Autodesk Inventor part; units mm, degrees
(part 2 of 2)
sketch "Sketch9" plane through (0, 0, 5.08) normal (0, 0, 1) x (1, 0, 0)
  arc A0 (133.35, 41.728) -> (148.59, 41.728) centre (140.97, 41.728) ccw projected
  line L0 (133.35, 41.728) -> (133.35, 92.528) projected
  arc A1 (148.59, 92.528) -> (133.35, 92.528) centre (140.97, 92.528) ccw projected
  line L1 (148.59, 92.528) -> (148.59, 41.728) projected
  line L2 (104.14, 0) -> (104.14, 5.08) projected
  line L3 (104.14, 5.08) -> (114.3, 5.08) projected
  line L4 (114.3, 5.08) -> (114.3, 0) projected
  line L5 (114.3, 0) -> (104.14, 0) projected
  line L6 (93.98, 5.08) -> (93.98, 0) projected
  line L7 (93.98, 0) -> (83.82, 0) projected
  line L8 (83.82, 0) -> (83.82, 5.08) projected
  line L9 (83.82, 5.08) -> (93.98, 5.08) projected
  line L10 (124.46, 0) -> (124.46, 5.08) projected
  line L11 (124.46, 5.08) -> (134.62, 5.08) projected
  line L12 (134.62, 5.08) -> (134.62, 0) projected
  line L13 (134.62, 0) -> (124.46, 0) projected
  line L14 (157.48, 65.405) -> (157.48, 55.245) projected
  line L15 (157.48, 55.245) -> (152.4, 55.245) projected
  line L16 (152.4, 55.245) -> (152.4, 65.405) projected
  line L17 (152.4, 65.405) -> (157.48, 65.405) projected
  line L18 (157.48, 45.085) -> (157.48, 34.925) projected
  line L19 (157.48, 34.925) -> (152.4, 34.925) projected
  line L20 (152.4, 34.925) -> (152.4, 45.085) projected
  line L21 (152.4, 45.085) -> (157.48, 45.085) projected
  line L22 (157.48, 24.765) -> (157.48, 14.605) projected
  line L23 (157.48, 14.605) -> (152.4, 14.605) projected
  line L24 (152.4, 14.605) -> (152.4, 24.765) projected
  line L25 (152.4, 24.765) -> (157.48, 24.765) projected
  line L26 (30.48, -80.01) -> (30.48, -90.17) projected
  line L27 (30.48, -90.17) -> (25.4, -90.17) projected
  line L28 (25.4, -90.17) -> (25.4, -80.01) projected
  line L29 (25.4, -80.01) -> (30.48, -80.01) projected
  line L30 (25.4, -59.69) -> (30.48, -59.69) projected
  line L31 (30.48, -59.69) -> (30.48, -69.85) projected
  line L32 (30.48, -69.85) -> (25.4, -69.85) projected
  line L33 (25.4, -69.85) -> (25.4, -59.69) projected
  line L34 (25.4, -39.37) -> (30.48, -39.37) projected
  line L35 (30.48, -39.37) -> (30.48, -49.53) projected
  line L36 (30.48, -49.53) -> (25.4, -49.53) projected
  line L37 (25.4, -49.53) -> (25.4, -39.37) projected
  line L38 (129.54, 45.72) -> (124.46, 45.72) projected
  line L39 (124.46, 45.72) -> (124.46, 55.88) projected
  line L40 (124.46, 55.88) -> (129.54, 55.88) projected
  line L41 (129.54, 55.88) -> (129.54, 45.72) projected
  line L42 (129.54, 96.52) -> (129.54, 86.36) projected
  line L43 (129.54, 86.36) -> (124.46, 86.36) projected
  line L44 (124.46, 86.36) -> (124.46, 96.52) projected
  line L45 (124.46, 96.52) -> (129.54, 96.52) projected
  line L46 (129.54, 76.2) -> (129.54, 66.04) projected
  line L47 (129.54, 66.04) -> (124.46, 66.04) projected
  line L48 (124.46, 66.04) -> (124.46, 76.2) projected
  line L49 (124.46, 76.2) -> (129.54, 76.2) projected
  line L50 (129.54, 111.578) -> (210.82, 111.578) projected
  line L51 (129.54, 111.578) -> (129.54, 106.68) projected
  line L52 (129.54, 106.68) -> (124.46, 106.68) projected
  line L53 (124.46, 106.68) -> (124.46, 111.578) projected
  line L54 (0, 111.578) -> (124.46, 111.578) projected
  line L55 (0, 111.578) -> (0, 101.6) projected
  line L56 (0, 101.6) -> (5.08, 101.6) projected
  line L57 (5.08, 101.6) -> (5.08, 91.44) projected
  line L58 (5.08, 91.44) -> (0, 91.44) projected
  line L59 (0, 91.44) -> (0, 81.28) projected
  line L60 (0, 81.28) -> (5.08, 81.28) projected
  line L61 (5.08, 81.28) -> (5.08, 71.12) projected
  line L62 (5.08, 71.12) -> (0, 71.12) projected
  line L63 (0, 71.12) -> (0, 60.96) projected
  line L64 (0, 60.96) -> (5.08, 60.96) projected
  line L65 (5.08, 60.96) -> (5.08, 50.8) projected
  line L66 (5.08, 50.8) -> (0, 50.8) projected
  line L67 (0, 50.8) -> (0, 40.64) projected
  line L68 (0, 40.64) -> (5.08, 40.64) projected
  line L69 (5.08, 40.64) -> (5.08, 30.48) projected
  line L70 (5.08, 30.48) -> (0, 30.48) projected
  line L71 (0, 30.48) -> (0, 20.32) projected
  line L72 (0, 20.32) -> (5.08, 20.32) projected
  line L73 (5.08, 20.32) -> (5.08, 10.16) projected
  line L74 (5.08, 10.16) -> (0, 10.16) projected
  line L75 (0, 10.16) -> (0, 0) projected
  line L76 (0, 0) -> (20.32, -95.25) projected
  line L77 (20.32, -95.25) -> (42.545, -95.25) projected
  line L78 (42.545, -95.25) -> (147.32, 9.525) projected
  line L79 (147.32, 9.525) -> (169.545, 9.525) projected
  line L80 (169.545, 9.525) -> (215.9, 35.56) projected
  line L81 (215.9, 35.56) -> (215.9, 45.72) projected
  line L82 (215.9, 45.72) -> (210.82, 45.72) projected
  line L83 (210.82, 45.72) -> (210.82, 55.88) projected
  line L84 (210.82, 55.88) -> (215.9, 55.88) projected
  line L85 (215.9, 55.88) -> (215.9, 66.04) projected
  line L86 (215.9, 66.04) -> (210.82, 66.04) projected
  line L87 (210.82, 66.04) -> (210.82, 76.2) projected
  line L88 (210.82, 76.2) -> (215.9, 76.2) projected
  line L89 (215.9, 76.2) -> (215.9, 86.36) projected
  line L90 (215.9, 86.36) -> (210.82, 86.36) projected
  line L91 (210.82, 86.36) -> (210.82, 96.52) projected
  line L92 (210.82, 96.52) -> (215.9, 96.52) projected
  line L93 (215.9, 96.52) -> (215.9, 106.68) projected
  line L94 (215.9, 106.68) -> (210.82, 106.68) projected
  line L95 (210.82, 106.68) -> (210.82, 111.578) projected
  line L96 (140.97, 92.528) -> (185.42, 92.528) construction
  line L97 (140.97, 84.908) -> (185.42, 84.908)
  line L98 (185.42, 100.148) -> (140.97, 100.148)
  arc A2 (140.97, 100.148) -> (140.97, 84.908) centre (140.97, 92.528) ccw
  arc A3 (185.42, 84.908) -> (185.42, 100.148) centre (185.42, 92.528) ccw
  point P0 (163.195, 92.528)
  dimension "d79" = 44.45
  dimension "d83" = 7.62
  constraints: 8 end point, 4 point on circle, 4 tangent, 2 centre point, 1 horizontal, 1 midpoint, 1 parallel
  measures "d79" distance of L96.start L96.end
  measures "d83" radius of A2
extrude "Extrusion10" cut sketch "Sketch9" against normal blind 25.4 contours A1 L1 L97 A2 | L1 A1 L98 A3 L97
fillet "Fillet1" radius 7.62 1 edges at (148.59, 84.908, 2.54)
sketch "Sketch10" plane through (0, 0, 5.08) normal (0, 0, 1) x (1, 0, 0)
  arc A0 (156.21, 84.908) -> (148.59, 77.288) centre (156.21, 77.288) ccw projected
  line L0 (148.59, 77.288) -> (148.59, 41.728) projected
  arc A1 (133.35, 41.728) -> (148.59, 41.728) centre (140.97, 41.728) ccw projected
  line L1 (133.35, 41.728) -> (133.35, 92.528) projected
  arc A2 (140.97, 100.148) -> (133.35, 92.528) centre (140.97, 92.528) ccw projected
  line L2 (140.97, 100.148) -> (185.42, 100.148) projected
  arc A3 (185.42, 84.908) -> (185.42, 100.148) centre (185.42, 92.528) ccw projected
  line L3 (185.42, 84.908) -> (156.21, 84.908) projected
  line L4 (129.54, 111.578) -> (210.82, 111.578) projected
  line L5 (129.54, 111.578) -> (129.54, 106.68) projected
  line L6 (129.54, 106.68) -> (124.46, 106.68) projected
  line L7 (124.46, 106.68) -> (124.46, 111.578) projected
  line L8 (0, 111.578) -> (124.46, 111.578) projected
  line L9 (0, 111.578) -> (0, 101.6) projected
  line L10 (0, 101.6) -> (5.08, 101.6) projected
  line L11 (5.08, 101.6) -> (5.08, 91.44) projected
  line L12 (5.08, 91.44) -> (0, 91.44) projected
  line L13 (0, 91.44) -> (0, 81.28) projected
  line L14 (0, 81.28) -> (5.08, 81.28) projected
  line L15 (5.08, 81.28) -> (5.08, 71.12) projected
  line L16 (5.08, 71.12) -> (0, 71.12) projected
  line L17 (0, 71.12) -> (0, 60.96) projected
  line L18 (0, 60.96) -> (5.08, 60.96) projected
  line L19 (5.08, 60.96) -> (5.08, 50.8) projected
  line L20 (5.08, 50.8) -> (0, 50.8) projected
  line L21 (0, 50.8) -> (0, 40.64) projected
  line L22 (0, 40.64) -> (5.08, 40.64) projected
  line L23 (5.08, 40.64) -> (5.08, 30.48) projected
  line L24 (5.08, 30.48) -> (0, 30.48) projected
  line L25 (0, 30.48) -> (0, 20.32) projected
  line L26 (0, 20.32) -> (5.08, 20.32) projected
  line L27 (5.08, 20.32) -> (5.08, 10.16) projected
  line L28 (5.08, 10.16) -> (0, 10.16) projected
  line L29 (0, 10.16) -> (0, 0) projected
  line L30 (0, 0) -> (20.32, -95.25) projected
  line L31 (20.32, -95.25) -> (42.545, -95.25) projected
  line L32 (42.545, -95.25) -> (147.32, 9.525) projected
  line L33 (147.32, 9.525) -> (169.545, 9.525) projected
  line L34 (169.545, 9.525) -> (215.9, 35.56) projected
  line L35 (215.9, 35.56) -> (215.9, 45.72) projected
  line L36 (215.9, 45.72) -> (210.82, 45.72) projected
  line L37 (210.82, 45.72) -> (210.82, 55.88) projected
  line L38 (210.82, 55.88) -> (215.9, 55.88) projected
  line L39 (215.9, 55.88) -> (215.9, 66.04) projected
  line L40 (215.9, 66.04) -> (210.82, 66.04) projected
  line L41 (210.82, 66.04) -> (210.82, 76.2) projected
  line L42 (210.82, 76.2) -> (215.9, 76.2) projected
  line L43 (215.9, 76.2) -> (215.9, 86.36) projected
  line L44 (215.9, 86.36) -> (210.82, 86.36) projected
  line L45 (210.82, 86.36) -> (210.82, 96.52) projected
  line L46 (210.82, 96.52) -> (215.9, 96.52) projected
  line L47 (215.9, 96.52) -> (215.9, 106.68) projected
  line L48 (215.9, 106.68) -> (210.82, 106.68) projected
  line L49 (210.82, 106.68) -> (210.82, 111.578) projected
  line L50 (129.54, 76.2) -> (129.54, 66.04) projected
  line L51 (129.54, 66.04) -> (124.46, 66.04) projected
  line L52 (124.46, 66.04) -> (124.46, 76.2) projected
  line L53 (124.46, 76.2) -> (129.54, 76.2) projected
  line L54 (129.54, 96.52) -> (129.54, 86.36) projected
  line L55 (129.54, 86.36) -> (124.46, 86.36) projected
  line L56 (124.46, 86.36) -> (124.46, 96.52) projected
  line L57 (124.46, 96.52) -> (129.54, 96.52) projected
  line L58 (129.54, 45.72) -> (124.46, 45.72) projected
  line L59 (124.46, 45.72) -> (124.46, 55.88) projected
  line L60 (124.46, 55.88) -> (129.54, 55.88) projected
  line L61 (129.54, 55.88) -> (129.54, 45.72) projected
  line L62 (25.4, -39.37) -> (30.48, -39.37) projected
  line L63 (30.48, -39.37) -> (30.48, -49.53) projected
  line L64 (30.48, -49.53) -> (25.4, -49.53) projected
  line L65 (25.4, -49.53) -> (25.4, -39.37) projected
  line L66 (25.4, -59.69) -> (30.48, -59.69) projected
  line L67 (30.48, -59.69) -> (30.48, -69.85) projected
  line L68 (30.48, -69.85) -> (25.4, -69.85) projected
  line L69 (25.4, -69.85) -> (25.4, -59.69) projected
  line L70 (30.48, -80.01) -> (30.48, -90.17) projected
  line L71 (30.48, -90.17) -> (25.4, -90.17) projected
  line L72 (25.4, -90.17) -> (25.4, -80.01) projected
  line L73 (25.4, -80.01) -> (30.48, -80.01) projected
  line L74 (157.48, 24.765) -> (157.48, 14.605) projected
  line L75 (157.48, 14.605) -> (152.4, 14.605) projected
  line L76 (152.4, 14.605) -> (152.4, 24.765) projected
  line L77 (152.4, 24.765) -> (157.48, 24.765) projected
  line L78 (157.48, 45.085) -> (157.48, 34.925) projected
  line L79 (157.48, 34.925) -> (152.4, 34.925) projected
  line L80 (152.4, 34.925) -> (152.4, 45.085) projected
  line L81 (152.4, 45.085) -> (157.48, 45.085) projected
  line L82 (157.48, 65.405) -> (157.48, 55.245) projected
  line L83 (157.48, 55.245) -> (152.4, 55.245) projected
  line L84 (152.4, 55.245) -> (152.4, 65.405) projected
  line L85 (152.4, 65.405) -> (157.48, 65.405) projected
  line L86 (124.46, 0) -> (124.46, 5.08) projected
  line L87 (124.46, 5.08) -> (134.62, 5.08) projected
  line L88 (134.62, 5.08) -> (134.62, 0) projected
  line L89 (134.62, 0) -> (124.46, 0) projected
  line L90 (93.98, 5.08) -> (93.98, 0) projected
  line L91 (93.98, 0) -> (83.82, 0) projected
  line L92 (83.82, 0) -> (83.82, 5.08) projected
  line L93 (83.82, 5.08) -> (93.98, 5.08) projected
  line L94 (104.14, 0) -> (104.14, 5.08) projected
  line L95 (104.14, 5.08) -> (114.3, 5.08) projected
  line L96 (114.3, 5.08) -> (114.3, 0) projected
  line L97 (114.3, 0) -> (104.14, 0) projected
  line L98 (38.1, 84.908) -> (38.1, 2.358) construction
  line L99 (22.86, 84.908) -> (22.86, 2.358)
  line L100 (53.34, 2.358) -> (53.34, 84.908)
  arc A4 (53.34, 84.908) -> (22.86, 84.908) centre (38.1, 84.908) ccw
  arc A5 (22.86, 2.358) -> (53.34, 2.358) centre (38.1, 2.358) ccw
  line L101 (160.02, 100.148) -> (23.9329, 100.148) construction
  line L102 (38.1, 84.908) -> (95.25, 84.908) construction
  line L103 (38.1, 69.668) -> (95.25, 69.668)
  line L104 (95.25, 100.148) -> (38.1, 100.148)
  arc A6 (38.1, 100.148) -> (38.1, 69.668) centre (38.1, 84.908) ccw
  arc A7 (95.25, 69.668) -> (95.25, 100.148) centre (95.25, 84.908) ccw
  point P0 (38.1, 43.633)
  point P1 (66.675, 84.908)
  dimension "d84" = 82.55
  dimension "d86" = 38.1
  dimension "d87" = 15.24
  dimension "d90" = 50.8
  dimension "d91" = 44.45
  dimension "d92" = 57.15
  dimension "d95" = 15.24
  dimension "d97" = 7.62
  constraints: 18 end point, 9 tangent, 8 point on circle, 4 centre point, 2 horizontal, 2 midpoint, 2 parallel, 1 concentric, 1 point on line, 1 vertical
  measures "d84" distance of L98.start L98.end
  measures "d86" distance between parallel lines of L9 L98
  measures "d87" radius of A5
  measures "d90" distance of A2.centre A1.centre
  measures "d91" distance of A3.centre A2.centre
  measures "d92" distance of L98.start L102.end
  measures "d95" radius of A6
  measures "d97" radius of A1
extrude "Extrusion11" cut sketch "Sketch10" against normal blind 25.4 contours A6 L103 L100 A5 L99 | A4 L100 L103 A6
extrude "Extrusion12" cut sketch "Sketch10" against normal blind 25.4 contours A4 L100 L103 A6 | L104 A7 L103 L100 A4
fillet "Fillet2" radius 15.24 1 edges at (53.34, 69.668, 2.54)
sketch "Sketch12" plane through (0, 0, 0) normal (0, 0, -1) x (-1, 0, 0)
  line L0 (-147.32, 9.525) -> (-42.545, -95.25) projected
  line L1 (-42.545, -95.25) -> (-20.32, -95.25) projected
  line L2 (-20.32, -95.25) -> (0, 0) projected
  line L3 (0, 10.16) -> (0, 0) projected
  line L4 (0, 10.16) -> (-5.08, 10.16) projected
  line L5 (-5.08, 10.16) -> (-5.08, 20.32) projected
  line L6 (-5.08, 20.32) -> (0, 20.32) projected
  line L7 (0, 30.48) -> (0, 20.32) projected
  line L8 (0, 30.48) -> (-5.08, 30.48) projected
  line L9 (-5.08, 30.48) -> (-5.08, 40.64) projected
  line L10 (-5.08, 40.64) -> (0, 40.64) projected
  line L11 (0, 50.8) -> (0, 40.64) projected
  line L12 (0, 50.8) -> (-5.08, 50.8) projected
  line L13 (-5.08, 50.8) -> (-5.08, 60.96) projected
  line L14 (-5.08, 60.96) -> (0, 60.96) projected
  line L15 (0, 71.12) -> (0, 60.96) projected
  line L16 (0, 71.12) -> (-5.08, 71.12) projected
  line L17 (-5.08, 71.12) -> (-5.08, 81.28) projected
  line L18 (-5.08, 81.28) -> (0, 81.28) projected
  line L19 (0, 91.44) -> (0, 81.28) projected
  line L20 (0, 91.44) -> (-5.08, 91.44) projected
  line L21 (-5.08, 91.44) -> (-5.08, 101.6) projected
  line L22 (-5.08, 101.6) -> (0, 101.6) projected
  line L23 (0, 111.578) -> (0, 101.6) projected
  line L24 (-124.46, 111.578) -> (0, 111.578) projected
  line L25 (-124.46, 111.578) -> (-124.46, 106.68) projected
  line L26 (-124.46, 106.68) -> (-129.54, 106.68) projected
  line L27 (-129.54, 106.68) -> (-129.54, 111.578) projected
  line L28 (-210.82, 111.578) -> (-129.54, 111.578) projected
  line L29 (-210.82, 111.578) -> (-210.82, 106.68) projected
  line L30 (-210.82, 106.68) -> (-215.9, 106.68) projected
  line L31 (-215.9, 106.68) -> (-215.9, 96.52) projected
  line L32 (-215.9, 96.52) -> (-210.82, 96.52) projected
  line L33 (-210.82, 96.52) -> (-210.82, 86.36) projected
  line L34 (-210.82, 86.36) -> (-215.9, 86.36) projected
  line L35 (-215.9, 86.36) -> (-215.9, 76.2) projected
  line L36 (-215.9, 76.2) -> (-210.82, 76.2) projected
  line L37 (-210.82, 76.2) -> (-210.82, 66.04) projected
  line L38 (-210.82, 66.04) -> (-215.9, 66.04) projected
  line L39 (-215.9, 66.04) -> (-215.9, 55.88) projected
  line L40 (-215.9, 55.88) -> (-210.82, 55.88) projected
  line L41 (-210.82, 55.88) -> (-210.82, 45.72) projected
  line L42 (-210.82, 45.72) -> (-215.9, 45.72) projected
  line L43 (-215.9, 45.72) -> (-215.9, 35.56) projected
  line L44 (-215.9, 35.56) -> (-169.545, 9.525) projected
  line L45 (-169.545, 9.525) -> (-147.32, 9.525) projected
  arc A0 (-148.59, 77.288) -> (-156.21, 84.908) centre (-156.21, 77.288) ccw projected
  line L46 (-156.21, 84.908) -> (-185.42, 84.908) projected
  arc A1 (-185.42, 100.148) -> (-185.42, 84.908) centre (-185.42, 92.528) ccw projected
  line L47 (-185.42, 100.148) -> (-140.97, 100.148) projected
  arc A2 (-133.35, 92.528) -> (-140.97, 100.148) centre (-140.97, 92.528) ccw projected
  line L48 (-133.35, 92.528) -> (-133.35, 41.728) projected
  arc A3 (-148.59, 41.728) -> (-133.35, 41.728) centre (-140.97, 41.728) ccw projected
  line L49 (-148.59, 41.728) -> (-148.59, 77.288) projected
  line L50 (-104.14, 5.08) -> (-104.14, 0) projected
  line L51 (-104.14, 0) -> (-114.3, 0) projected
  line L52 (-114.3, 0) -> (-114.3, 5.08) projected
  line L53 (-114.3, 5.08) -> (-104.14, 5.08) projected
  line L54 (-93.98, 0) -> (-93.98, 5.08) projected
  line L55 (-93.98, 5.08) -> (-83.82, 5.08) projected
  line L56 (-83.82, 5.08) -> (-83.82, 0) projected
  line L57 (-83.82, 0) -> (-93.98, 0) projected
  line L58 (-124.46, 5.08) -> (-124.46, 0) projected
  line L59 (-124.46, 0) -> (-134.62, 0) projected
  line L60 (-134.62, 0) -> (-134.62, 5.08) projected
  line L61 (-134.62, 5.08) -> (-124.46, 5.08) projected
  line L62 (-157.48, 55.245) -> (-157.48, 65.405) projected
  line L63 (-157.48, 65.405) -> (-152.4, 65.405) projected
  line L64 (-152.4, 65.405) -> (-152.4, 55.245) projected
  line L65 (-152.4, 55.245) -> (-157.48, 55.245) projected
  line L66 (-157.48, 34.925) -> (-157.48, 45.085) projected
  line L67 (-157.48, 45.085) -> (-152.4, 45.085) projected
  line L68 (-152.4, 45.085) -> (-152.4, 34.925) projected
  line L69 (-152.4, 34.925) -> (-157.48, 34.925) projected
  line L70 (-157.48, 14.605) -> (-157.48, 24.765) projected
  line L71 (-157.48, 24.765) -> (-152.4, 24.765) projected
  line L72 (-152.4, 24.765) -> (-152.4, 14.605) projected
  line L73 (-152.4, 14.605) -> (-157.48, 14.605) projected
  line L74 (-30.48, -90.17) -> (-30.48, -80.01) projected
  line L75 (-30.48, -80.01) -> (-25.4, -80.01) projected
  line L76 (-25.4, -80.01) -> (-25.4, -90.17) projected
  line L77 (-25.4, -90.17) -> (-30.48, -90.17) projected
  line L78 (-30.48, -59.69) -> (-25.4, -59.69) projected
  line L79 (-25.4, -59.69) -> (-25.4, -69.85) projected
  line L80 (-25.4, -69.85) -> (-30.48, -69.85) projected
  line L81 (-30.48, -69.85) -> (-30.48, -59.69) projected
  line L82 (-30.48, -39.37) -> (-25.4, -39.37) projected
  line L83 (-25.4, -39.37) -> (-25.4, -49.53) projected
  line L84 (-25.4, -49.53) -> (-30.48, -49.53) projected
  line L85 (-30.48, -49.53) -> (-30.48, -39.37) projected
  line L86 (-124.46, 45.72) -> (-129.54, 45.72) projected
  line L87 (-129.54, 45.72) -> (-129.54, 55.88) projected
  line L88 (-129.54, 55.88) -> (-124.46, 55.88) projected
  line L89 (-124.46, 55.88) -> (-124.46, 45.72) projected
  line L90 (-129.54, 86.36) -> (-129.54, 96.52) projected
  line L91 (-129.54, 96.52) -> (-124.46, 96.52) projected
  line L92 (-124.46, 96.52) -> (-124.46, 86.36) projected
  line L93 (-124.46, 86.36) -> (-129.54, 86.36) projected
  line L94 (-129.54, 66.04) -> (-129.54, 76.2) projected
  line L95 (-129.54, 76.2) -> (-124.46, 76.2) projected
  line L96 (-124.46, 76.2) -> (-124.46, 66.04) projected
  line L97 (-124.46, 66.04) -> (-129.54, 66.04) projected
  arc A4 (-53.34, 54.428) -> (-68.58, 69.668) centre (-68.58, 54.428) ccw projected
  line L98 (-68.58, 69.668) -> (-95.25, 69.668) projected
  arc A5 (-95.25, 100.148) -> (-95.25, 69.668) centre (-95.25, 84.908) ccw projected
  line L99 (-95.25, 100.148) -> (-38.1, 100.148) projected
  arc A6 (-22.86, 84.908) -> (-38.1, 100.148) centre (-38.1, 84.908) ccw projected
  line L100 (-22.86, 84.908) -> (-22.86, 2.358) projected
  arc A7 (-53.34, 2.358) -> (-22.86, 2.358) centre (-38.1, 2.358) ccw projected
  line L101 (-53.34, 2.358) -> (-53.34, 54.428) projected
  line L102 (-93.8352, -43.9598) -> (-86.651, -51.144)
  line L103 (-86.651, -51.144) -> (-83.0589, -47.5519)
  line L104 (-83.0589, -47.5519) -> (-90.2431, -40.3677)
  line L105 (-90.2431, -40.3677) -> (-93.8352, -43.9598)
  line L106 (-136.9405, -0.8545) -> (-129.7563, -8.0387)
  line L107 (-129.7563, -8.0387) -> (-126.1642, -4.4466)
  line L108 (-126.1642, -4.4466) -> (-133.3484, 2.7376)
  line L109 (-133.3484, 2.7376) -> (-136.9405, -0.8545)
  dimension "d102" = 10.16
  dimension "d104" = 5.08
  constraints: 16 end point, 4 parallel, 2 perpendicular
  measures "d102" distance of L103.end L104.end
  measures "d104" distance of L102.end L103.end
sketch "Sketch13" plane through (0, 0, 0) normal (0, 0, -1) x (-1, 0, 0)
  line L0 (-125.7393, -12.0557) -> (-118.5551, -19.2399)
  line L1 (-118.5551, -19.2399) -> (-114.963, -15.6478)
  line L2 (-114.963, -15.6478) -> (-122.1472, -8.4636)
  line L3 (-122.1472, -8.4636) -> (-125.7393, -12.0557)
  line L4 (-147.32, 9.525) -> (-42.545, -95.25) projected
  line L5 (-124.46, 0) -> (-131.1275, -6.6675) construction
  line L6 (-111.3709, -26.4241) -> (-104.1867, -33.6083)
  line L7 (-104.1867, -33.6083) -> (-100.5946, -30.0162)
  line L8 (-100.5946, -30.0162) -> (-107.7788, -22.832)
  line L9 (-107.7788, -22.832) -> (-111.3709, -26.4241)
  line L10 (-97.0025, -40.7925) -> (-89.8183, -47.9767)
  line L11 (-89.8183, -47.9767) -> (-86.2262, -44.3846)
  line L12 (-86.2262, -44.3846) -> (-93.4104, -37.2004)
  line L13 (-93.4104, -37.2004) -> (-97.0025, -40.7925)
  point P0 (0, 0)
  point P1 (-124.46, 0)
  dimension "d110" = 5.08
  dimension "d111" = 10.16
  dimension "d112" = 7.62
  dimension "d115" = 20.32
  constraints: 26 end point, 2 parallel, 2 perpendicular, 1 coincident, 1 collinear, 1 point on line, 17 other
  measures "d110" distance of L0.end L1.end
  measures "d111" distance of L1.end L2.end
  measures "d112" distance between parallel lines of L3 L5
  measures "d115" distance of L0.start L6.start
extrude "Extrusion16" cut sketch "Sketch13" against normal blind 5.08
sketch "Sketch14" plane through (0, 0, 0) normal (0, 0, -1) x (-1, 0, 0)
  line L0 (-89.8183, -47.9767) -> (-42.545, -95.25) projected
  line L1 (-89.8183, -47.9767) -> (-82.6341, -55.1609)
  line L2 (-82.6341, -55.1609) -> (-79.042, -51.5688)
  line L3 (-79.042, -51.5688) -> (-86.2262, -44.3846)
  line L4 (-86.2262, -44.3846) -> (-89.8183, -47.9767)
  line L5 (-125.7393, -12.0557) -> (-147.32, 9.525) projected
  line L6 (-125.7393, -12.0557) -> (-132.9236, -4.8714)
  line L7 (-132.9236, -4.8714) -> (-129.3314, -1.2793)
  line L8 (-129.3314, -1.2793) -> (-122.1472, -8.4636)
  line L9 (-122.1472, -8.4636) -> (-125.7393, -12.0557)
  line L10 (-125.7393, -12.0557) -> (-122.1472, -8.4636) projected
  point P0 (0, 0)
  dimension "d122" = 10.16
  dimension "d123" = 5.08
  dimension "d124" = 10.16
  dimension "d125" = 5.08
  constraints: 16 end point, 4 parallel, 2 perpendicular, 2 point on line, 1 collinear
  measures "d122" distance of L0.start L1.end
  measures "d123" distance of L2.end L1.end
  measures "d124" distance of L6.start L6.end
  measures "d125" distance of L6.end L7.end
equation "\"d4\" = d3"
equation "\"d7\" = 2 * d3"
equation "\"d22\" = d99"
equation "\"d29\" = d27"
equation "\"d65\" = 2 * d59"
equation "\"d74\" = 0.5 * d73"
body "Solid2"
